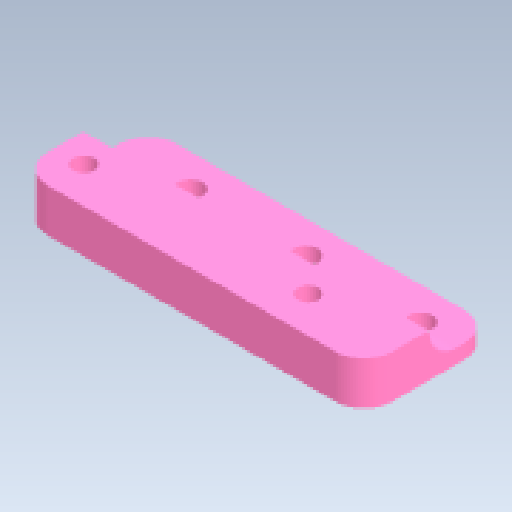
# Autodesk Inventor part: DriveMotorMount5
Saved by Autodesk Inventor 2023 (Build 270158000, 158)
## iProperties
Created: 2023-04-07
Part Number: DriveMotorMount5
Material: Generic
Document SubType Name: Modeling
Designer: Dave
Density: 1 g/cm^3
Appearance: Pink
Author: Dave
Autodesk Inventor part; units mm, degrees
ref_plane "YZ Plane" through (0, 0, 0) normal (1, 0, 0) x (0, 1, 0)
ref_plane "XZ Plane" through (0, 0, 0) normal (0, 1, 0) x (-1, 0, 0)
ref_plane "XY Plane" through (0, 0, 0) normal (0, 0, 1) x (1, 0, 0)
sketch "Sketch1" plane through (0, 0, 0) normal (1, 0, 0) x (0, 1, 0)
  line L0 (0, 0) -> (0, -28.575)
  line L1 (0, -28.575) -> (3.175, -28.575)
  line L2 (3.175, -28.575) -> (3.175, -14.2875)
  line L3 (3.175, -14.2875) -> (9.525, -14.2875)
  line L4 (9.525, -14.2875) -> (9.525, 0)
  line L5 (9.525, 0) -> (0, 0)
  point P0 (0, -14.2875)
  dimension "d0" = 3.175
  dimension "d1" = 9.525
  dimension "d2" = 28.575
  constraints: 12 end point, 5 perpendicular, 1 horizontal alignment, 1 midpoint, 1 vertical
  measures "d0" distance of L0.end L1.end
  measures "d1" distance of L4.end L0.start
  measures "d2" distance of L0.start L0.end
extrude "Extrusion1" add sketch "Sketch1" along normal blind 76.2
sketch "Sketch2" plane through (0, 9.525, 0) normal (0, 1, 0) x (1, 0, 0)
  circle A0 centre (16.5354, 21.3995) radius 2.65
  circle A1 centre (41.9354, 21.3995) radius 2.65
  circle A2 centre (67.3354, 21.3995) radius 2.65
  circle A3 centre (55.8475, 8.0391) radius 2.25
  circle A4 centre (6.35, 8.0391) radius 2.25
  line L0 (0, 28.575) -> (0, 14.2875) projected
  line L1 (0, 14.2875) -> (0, 0) projected
  line L2 (0, 14.2875) -> (76.2, 14.2875) projected
  point P0 (0, 21.4313)
  point P1 (0, 7.1438)
  dimension "d5" = 5.3
  dimension "d6" = 25.4
  dimension "d7" = 25.4
  dimension "d8" = 49.4975
  dimension "d9" = 4.5
  dimension "d10" = 13.3604
  dimension "d11" = 10.1854
  dimension "d13" = 7.112
  dimension "d14" = 6.35
  constraints: 5 centre point, 3 equal radius, 3 horizontal alignment, 2 midpoint
  measures "d5" diameter of A0
  measures "d6" distance of A0.centre A1.centre
  measures "d7" distance of A1.centre A2.centre
  measures "d8" distance of A3.centre A4.centre
  measures "d9" diameter of A4
  measures "d10" vertical distance of A4.centre A0.centre
  measures "d11" horizontal distance of A0.centre A4.centre
  measures "d13" distance from line of L2 A0.centre
  measures "d14" distance from line of L1 A4.centre
extrude "Extrusion2" cut sketch "Sketch2" against normal through all
sketch "Sketch3" plane through (0, 0, -28.575) normal (0, -1, 0) x (1, 0, 0)
  circle A0 centre (55.8475, 20.5359) radius 2.25 projected
  circle A1 centre (55.8475, 20.5359) radius 2.625
  circle A2 centre (6.35, 20.5359) radius 2.25 projected
  circle A3 centre (6.35, 20.5359) radius 2.625
  point P0 (0, 28.575)
  dimension "d17" = 5.25
  dimension "d18" = 5.25
  constraints: 2 centre point, 2 coincident
  measures "d17" diameter of A1
  measures "d18" diameter of A3
extrude "Extrusion3" cut sketch "Sketch3" against normal blind 5
fillet "Fillet1" radius 6.35 5 edges at (76.2, 4.7625, 0) (38.1, 3.175, -14.2875) (76.2, 1.5875, -28.575) (0, 1.5875, -28.575) (0, 4.7625, 0)
equation "\"d7\" = d6"
body "Solid1"
